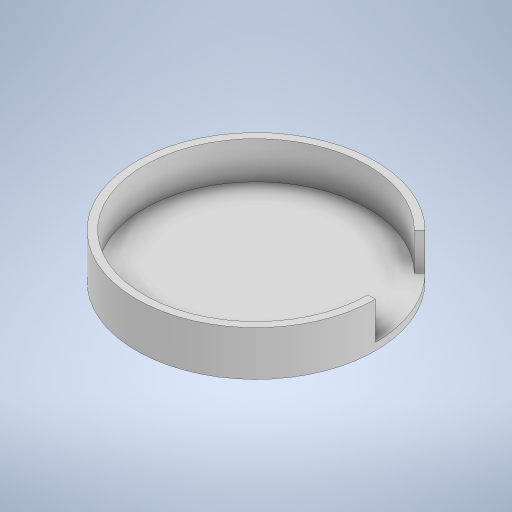
# Autodesk Inventor part: mainbody
Saved by Autodesk Inventor 2024 (Build 280153000, 153)
## iProperties
Created: 2024-05-20
Part Number: mainbody
Material: Generic
Document SubType Name: Modeling
Designer: ryana
Density: 1 g/cm^3
Appearance: Default
Author: ryana
Autodesk Inventor part; units mm, degrees
ref_plane "YZ Plane" through (0, 0, 0) normal (1, 0, 0) x (0, 1, 0)
ref_plane "XZ Plane" through (0, 0, 0) normal (0, 1, 0) x (-1, 0, 0)
ref_plane "XY Plane" through (0, 0, 0) normal (0, 0, 1) x (1, 0, 0)
sketch "Sketch1" plane through (0, 0, 0) normal (0, 1, 0) x (-1, 0, 0)
  circle A0 centre (0, 0) radius 45
  circle A1 centre (0, 0) radius 48
  dimension "d0" = 90
  dimension "d1" = 96
  constraints: 2 centre point, 2 coincident
  measures "d0" diameter of A0
  measures "d1" diameter of A1
extrude "Extrusion3" add sketch "Sketch1" along normal blind 18
sketch "Sketch3" plane through (0, 0, 0) normal (0, 1, 0) x (-1, 0, 0)
  circle A0 centre (0, 0) radius 45
  dimension "d9" = 90
  constraints: 1 centre point, 1 coincident
  measures "d9" diameter of A0
extrude "Extrusion4" add sketch "Sketch3" along normal blind 3
sketch "Sketch4" plane through (0, 3, 0) normal (0, 1, 0) x (1, 0, 0)
  line L0 (0, 0) -> (48, 0)
  line L1 (0, 0) -> (48, 0) construction
  line L2 (0, 0) -> (33.9411, 33.9411)
  line L3 (0, 0) -> (48, 0) construction
  arc A0 (48, 0) -> (33.9411, 33.9411) centre (0, 0) ccw
  dimension "d12" = 48
  dimension "d13" = 0
  dimension "d14" = 48
  dimension "d15" = 45
  dimension "d16" = 48
  constraints: 8 end point, 3 horizontal, 2 equal length, 2 point on circle, 1 centre point
  measures "d12" distance of L0.start L0.end
  measures "d13" distance between parallel lines of L0 L1
  measures "d14" distance of L0.start L2.end
  measures "d15" angle of L3 L2
  measures "d16" radius of A0
extrude "Extrusion5" cut sketch "Sketch4" along normal blind 20
body "Solid2"
